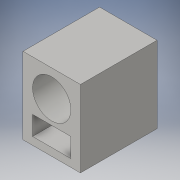
# Autodesk Inventor part: Pivot Poin 3
Saved by Autodesk Inventor 2016 (Build 200138000, 138)
## iProperties
Created: 2016-03-19
Part Number: Pivot Poin 3
Material: Generic
Document SubType Name: Modeling
Designer: matth_000
Density: 1 g/cm^3
Appearance: Default
Author: matth_000
Autodesk Inventor part; units mm, degrees
ref_plane "YZ Plane" through (0, 0, 0) normal (1, 0, 0) x (0, 1, 0)
ref_plane "XZ Plane" through (0, 0, 0) normal (0, 1, 0) x (-1, 0, 0)
ref_plane "XY Plane" through (0, 0, 0) normal (0, 0, 1) x (1, 0, 0)
sketch "Sketch1" plane through (0, 0, 0) normal (0, 1, 0) x (-1, 0, 0)
  line L0 (0, 0) -> (19.05, 0)
  line L1 (19.05, 0) -> (19.05, -25.4)
  line L2 (19.05, -25.4) -> (0, -25.4)
  line L3 (0, -25.4) -> (0, 0)
  dimension "d0" = 19.05
  dimension "d1" = 25.4
  constraints: 8 end point, 2 parallel, 1 horizontal, 1 perpendicular
  measures "d0" distance of L1.end L2.end
  measures "d1" distance of L0.end L1.end
extrude "Extrusion1" add sketch "Sketch1" along normal blind 25.4
sketch "Sketch2" plane through (-19.05, 0, 0) normal (0, 0, 1) x (1, 0, 0)
  circle A0 centre (9.525, 16.51) radius 6.35
  line L0 (0, 25.4) -> (19.05, 25.4) projected
  line L1 (3.175, 8.89) -> (15.875, 8.89)
  line L2 (15.875, 8.89) -> (15.875, 2.54)
  line L3 (15.875, 2.54) -> (3.175, 2.54)
  line L4 (3.175, 2.54) -> (3.175, 8.89)
  line L5 (0, 0) -> (0, 25.4) projected
  line L6 (19.05, 0) -> (19.05, 25.4) projected
  line L7 (19.05, 0) -> (0, 0) projected
  dimension "d4" = 12.7
  dimension "d5" = 8.89
  dimension "d6" = 12.7
  dimension "d7" = 19.05
  dimension "d8" = 6.35
  dimension "d9" = 3.175
  dimension "d10" = 3.175
  dimension "d16" = 2.54
  constraints: 8 end point, 2 parallel, 1 centre point, 1 horizontal, 1 perpendicular
  measures "d4" diameter of A0
  measures "d5" distance from line of L0 A0.centre
  measures "d6" distance of L2.end L3.end
  measures "d7" distance of L0.start L0.end
  measures "d8" distance of L3.end L1.start
  measures "d9" distance between parallel lines of L5 L4
  measures "d10" distance between parallel lines of L6 L2
  measures "d16" distance between parallel lines of L7 L3
extrude "Extrusion2" cut sketch "Sketch2" against normal blind 25.4 contours A0 | L1 L2 L3 L4
sketch "Sketch3" plane through (0, 0, 0) normal (0, -1, 0) x (1, 0, 0)
  circle A0 centre (-9.525, -12.7) radius 6.35
  point P0 (0, 0)
  dimension "d13" = 12.7
  constraints: 1 centre point
  measures "d13" diameter of A0
extrude "Extrusion3" cut sketch "Sketch3" against normal blind 3.175
body "Solid1"
